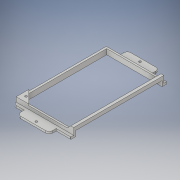
# Autodesk Inventor part: display_mount
Saved by Autodesk Inventor 2019 (Build 230136000, 136)
## iProperties
Created: 2021-12-03
Part Number: display_mount
Material: Generisch
Document SubType Name: Modeling
Designer: Bergi
Density: 1 g/cm^3
Appearance: Vorgabe
Author: Bergi
Autodesk Inventor part; units mm, degrees
ref_plane "YZ Plane" through (0, 0, 0) normal (1, 0, 0) x (0, 1, 0)
ref_plane "XZ Plane" through (0, 0, 0) normal (0, 1, 0) x (-1, 0, 0)
ref_plane "XY Plane" through (0, 0, 0) normal (0, 0, 1) x (1, 0, 0)
sketch "Skizze1" plane through (0, 0, 0) normal (0, 1, 0) x (-1, 0, 0)
  line L0 (-39, 60.5) -> (39, 60.5)
  line L1 (39, 60.5) -> (39, -60.5)
  line L2 (39, -60.5) -> (-39, -60.5)
  line L3 (-39, -60.5) -> (-39, 60.5)
  line L4 (-39, 60.5) -> (39, -60.5) construction
  line L5 (39, 60.5) -> (-39, -60.5) construction
  line L6 (42, 63.5) -> (-42, 63.5)
  line L7 (-42, 63.5) -> (-42, -63.5)
  line L8 (-42, -63.5) -> (42, -63.5)
  line L9 (42, -63.5) -> (42, 63.5)
  point P0 (0, 0)
  dimension "d0" = 78
  dimension "d1" = 121
  dimension "d2" = 3
  constraints: 20 end point, 4 parallel, 2 midpoint, 2 perpendicular, 1 horizontal, 3 other
  measures "d0" distance of L1.end L2.end
  measures "d1" distance of L0.end L1.end
  measures "d2" distance between parallel lines of L0 L6
extrude "Extrusion1" add sketch "Skizze1" along normal blind 7.5
sketch "Skizze2" plane through (0, 7.5, 0) normal (0, 1, 0) x (1, 0, 0)
  line L0 (39, -60.5) -> (-39, -60.5) projected
  line L1 (-39, -60.5) -> (-39, 60.5) projected
  circle A0 centre (-35.5, -56) radius 1.5
  point P0 (0, 0)
  dimension "d5" = 4.5
  dimension "d6" = 3.5
  dimension "d12" = 3
  constraints: 1 centre point, 1 coincident
  measures "d5" distance from line of L0 point (-35.5, -56)
  measures "d6" distance from line of L1 point (-35.5, -56)
  measures "d12" diameter of A0
sketch "Skizze3" plane through (0, 7.5, 0) normal (0, 1, 0) x (1, 0, 0)
  line L0 (-42, -63.5) -> (42, -63.5) projected
  line L1 (-42, -63.5) -> (-24, -63.5)
  line L2 (-42, -63.5) -> (-42, -45.5)
  line L3 (-42, 63.5) -> (-42, -63.5) projected
  line L4 (-42, -45.5) -> (-24, -63.5)
  point P0 (0, 0)
  dimension "d7" = 18
  dimension "d9" = 18
  constraints: 6 end point, 2 point on line
  measures "d7" distance of L0.start L1.end
  measures "d9" distance of L0.start L2.end
extrude "Extrusion2" add sketch "Skizze3" along normal blind 2
extrude "Extrusion3" cut sketch "Skizze2" along normal through all
ref_plane "Arbeitsebene1" through (0, 0, -60.5) normal (1, 0, 0) x (0, 0, -1)
ref_plane "Arbeitsebene2" through (39, 0, 0) normal (0, 0, -1) x (-1, 0, 0)
sketch "Skizze4" plane through (0, 0, 0) normal (0, -1, 0) x (1, 0, 0)
  line L0 (-39, -60.5) -> (-39, 60.5) projected
  line L1 (-39, 60.5) -> (39, 60.5) projected
  line L2 (39, 60.5) -> (39, -60.5) projected
  line L3 (39, -60.5) -> (-39, -60.5) projected
  line L4 (-42, 63.5) -> (42, 63.5) projected
  line L5 (-42, -63.5) -> (-42, 63.5) projected
  line L6 (42, -63.5) -> (-42, -63.5) projected
  line L7 (42, 63.5) -> (42, -63.5) projected
  line L8 (-42, 63.5) -> (42, 63.5) projected
  line L9 (-58.8, 0) -> (58.8, 0) construction
  line L10 (18.5, 63.5) -> (18.5, 72.5)
  line L11 (13.5, 77.5) -> (-21.5, 77.5)
  line L12 (-26.5, 72.5) -> (-26.5, 63.5)
  line L13 (42, 63.5) -> (42, 63.5)
  line L14 (38, 67.5) -> (-38, 67.5)
  line L15 (-42, 63.5) -> (-42, 63.5)
  line L16 (42, -63.5) -> (42, -63.5)
  line L17 (38, -67.5) -> (-38, -67.5)
  line L18 (-42, -63.5) -> (-42, -63.5)
  arc A0 (42, 63.5) -> (38, 67.5) centre (38, 63.5) ccw
  arc A1 (-38, 67.5) -> (-42, 63.5) centre (-38, 63.5) ccw
  arc A2 (-42, -63.5) -> (-38, -67.5) centre (-38, -63.5) ccw
  arc A3 (38, -67.5) -> (42, -63.5) centre (38, -63.5) ccw
  arc A4 (18.5, 72.5) -> (13.5, 77.5) centre (13.5, 72.5) ccw
  arc A5 (-21.5, 77.5) -> (-26.5, 72.5) centre (-21.5, 72.5) ccw
  line L19 (18.5, -63.5) -> (18.5, -72.5)
  line L20 (13.5, -77.5) -> (-21.5, -77.5)
  line L21 (-26.5, -72.5) -> (-26.5, -63.5)
  arc A6 (13.5, -77.5) -> (18.5, -72.5) centre (13.5, -72.5) ccw
  arc A7 (-26.5, -72.5) -> (-21.5, -77.5) centre (-21.5, -72.5) ccw
  line L22 (18.5, -63.5) -> (-26.5, -63.5)
  line L23 (42, -63.5) -> (-42, -63.5) projected
  line L24 (0, -109.9497) -> (0, 109.9497) construction
  point P0 (0, 0)
  point P1 (18.5, 77.5)
  point P2 (-26.5, 77.5)
  point P3 (-4, 77.5)
  point P4 (42, 67.5)
  point P5 (-42, 67.5)
  point P6 (42, -67.5)
  point P7 (-42, -67.5)
  point P8 (18.5, -77.5)
  point P9 (-26.5, -77.5)
  point P10 (-4, -77.5)
  point P11 (-4, 73)
  point P12 (-4, -73)
  dimension "d20" = 155
  dimension "d21" = 45
  dimension "d22" = 4
  dimension "d23" = 135
  dimension "d24" = 4
  dimension "d25" = 4
  dimension "d26" = 4
  dimension "d27" = 4
  dimension "d30" = 5
  dimension "d33" = 5.5
  constraints: 26 end point, 18 point on line, 16 point on circle, 14 symmetric about line, 12 tangent, 8 centre point, 5 perpendicular, 1 collinear, 1 equal radius, 1 midpoint, 1 vertical, 2 other
  measures "d20" diameter of L11 L9
  measures "d21" distance of point (18.5, 77.5) point (-26.5, 77.5)
  measures "d22" horizontal distance of point (0, 0) point (-4, 77.5)
  measures "d23" distance between parallel lines of L14 L17
  measures "d24" radius of A0
  measures "d25" radius of A1
  measures "d26" radius of A2
  measures "d27" radius of A3
  measures "d30" radius of A4
  measures "d33" distance from line of L14 point (-4, 73)
extrude "Extrusion4" add sketch "Skizze4" against normal blind 3 contours A1 L14 L12 L4 | L12 L14 L10 L4 | L6 L21 L17 A2 | L10 L14 A0 L4 | L6 L19 L17 L21 | L6 A3 L17 L19
extrude "Extrusion5" add sketch "Skizze4" against normal up to surface (3 mm away) contours L12 L14 L10 L4 | L12 A5 L11 A4 L10 L14 | L6 L19 L17 L21 | L17 L19 A6 L20 A7 L21
hole "Bohrung1" at (-4, 0, 73) at (-4, 0, -73) direction (0, 1, 0) diameter 3 end through all
sketch "Skizze6" plane through (42, 7.5, 63.5) normal (1, 0, 0) x (0, 0, -1)
  line L0 (0, -7.5) -> (127, -7.5) projected
  line L1 (127, -7.5) -> (127, -4.5) projected
  line L2 (127, -4.5) -> (127, 0) projected
  line L3 (0, 0) -> (127, 0) projected
  line L4 (0, -4.5) -> (0, 0) projected
  line L5 (0, -7.5) -> (0, -4.5) projected
  line L6 (131, -7.5) -> (127, -7.5) projected
  line L7 (131, -7.5) -> (131, -4.5) projected
  line L8 (127, -4.5) -> (131, -4.5) projected
  line L9 (127, -7.5) -> (127, -4.5) projected
  line L10 (0, -7.5) -> (-4, -7.5) projected
  line L11 (0, -7.5) -> (0, -4.5) projected
  line L12 (-4, -4.5) -> (0, -4.5) projected
  line L13 (-4, -7.5) -> (-4, -4.5) projected
  point P0 (63.5, -7.5)
extrude "Extrusion8" cut sketch "Skizze6" against normal up to surface (3 mm away)
sketch "Skizze7" plane through (0, 7.5, 0) normal (0, 1, 0) x (1, 0, 0)
  line L0 (39, -63.5) -> (39, -60.5) projected
  line L1 (39, -60.5) -> (-27, -60.5) projected
  line L2 (-27, -60.5) -> (-24, -63.5) projected
  line L3 (-24, -63.5) -> (39, -63.5) projected
  line L4 (39, 60.5) -> (39, 63.5) projected
  line L5 (39, 63.5) -> (-42, 63.5) projected
  line L6 (-42, 63.5) -> (-42, -45.5) projected
  line L7 (-42, -45.5) -> (-39, -48.5) projected
  line L8 (-39, -48.5) -> (-39, 60.5) projected
  line L9 (-39, 60.5) -> (39, 60.5) projected
  line L10 (39, -63.5) -> (39, 63.5)
  line L11 (39, 63.5) -> (-42, 63.5) projected
  line L12 (39, 63.5) -> (35, 63.5)
  line L13 (35, 63.5) -> (35, -63.5)
  line L14 (-42, -63.5) -> (39, -63.5) projected
  line L15 (35, -63.5) -> (39, -63.5)
  point P0 (0, 0)
  dimension "d48" = 4
  constraints: 8 end point, 2 collinear, 2 point on line, 1 perpendicular
  measures "d48" distance between parallel lines of L13 L10
extrude "Extrusion9" add sketch "Skizze7" along normal blind 5 contours L3 L13 L1 L0 | L1 L13 L9 L10 | L9 L13 L5 L4
sketch "Skizze8" plane through (-42, 3, -63.5) normal (0, 0, -1) x (-1, 0, 0)
  line L0 (-81, 9.5) -> (-81, 0) projected
  line L1 (-81, 0) -> (0, 0) projected
  line L2 (0, 0) -> (0, 4.5) projected
  line L3 (-77, 4.5) -> (0, 4.5) projected
  line L4 (-77, 4.5) -> (-77, 9.5) projected
  line L5 (-81, 9.5) -> (-77, 9.5) projected
  line L6 (-77, 4.5) -> (-77, 9.5) projected
  line L7 (-77, 9.5) -> (-72, 4.5)
  line L8 (-77, 4.5) -> (-15, 4.5) projected
  line L9 (-77, 9.5) -> (-69.9289, 9.5) construction
  line L10 (-72, 4.5) -> (-77, 4.5)
  line L11 (-77, 4.5) -> (-77, 9.5)
  point P0 (-42, -3)
  dimension "d51" = 45
  constraints: 8 end point, 1 collinear, 1 equal length, 1 horizontal, 1 perpendicular, 1 point on line
  measures "d51" angle of L7 L9
extrude "Extrusion10" add sketch "Skizze8" against normal up to surface (3 mm away) contours L7 L3 L4
sketch "Skizze9" plane through (-42, 9.5, 63.5) normal (0, 0, 1) x (1, 0, 0)
  line L0 (81, -9.5) -> (3, -9.5) projected
  line L1 (81, -9.5) -> (81, -2) projected
  line L2 (77, -2) -> (81, -2) projected
  line L3 (77, 3) -> (77, -2) projected
  line L4 (77, 3) -> (72, -2) projected
  line L5 (3, -2) -> (72, -2) projected
  line L6 (3, -9.5) -> (3, -2) projected
  line L7 (18, -2) -> (77, -2) projected
  line L8 (72, -2) -> (77, -2)
  point P0 (42, -9.5)
  constraints: 2 end point, 1 collinear
extrude "Extrusion11" add sketch "Skizze9" against normal up to surface (3 mm away) contours L7 L4 L3
sketch "Skizze10" plane through (0, 0, 0) normal (0, -1, 0) x (1, 0, 0)
  line L0 (39, -67.373) -> (39, -60.5) projected
  line L1 (39, -60.5) -> (-39, -60.5) projected
  line L2 (-39, -60.5) -> (-39, 60.5) projected
  line L3 (-39, 60.5) -> (39, 60.5) projected
  line L4 (39, 60.5) -> (39, 67.373) projected
  arc A0 (39, 67.373) -> (38, 67.5) centre (38, 63.5) ccw projected
  line L5 (38, 67.5) -> (18.5, 67.5) projected
  line L6 (18.5, 67.5) -> (18.5, 72.5) projected
  arc A1 (18.5, 72.5) -> (13.5, 77.5) centre (13.5, 72.5) ccw projected
  line L7 (13.5, 77.5) -> (-21.5, 77.5) projected
  arc A2 (-21.5, 77.5) -> (-26.5, 72.5) centre (-21.5, 72.5) ccw projected
  line L8 (-26.5, 72.5) -> (-26.5, 67.5) projected
  line L9 (-26.5, 67.5) -> (-38, 67.5) projected
  arc A3 (-38, 67.5) -> (-42, 63.5) centre (-38, 63.5) ccw projected
  line L10 (-42, -63.5) -> (-42, 63.5) projected
  arc A4 (-42, -63.5) -> (-38, -67.5) centre (-38, -63.5) ccw projected
  line L11 (-38, -67.5) -> (-26.5, -67.5) projected
  line L12 (-26.5, -67.5) -> (-26.5, -72.5) projected
  arc A5 (-26.5, -72.5) -> (-21.5, -77.5) centre (-21.5, -72.5) ccw projected
  line L13 (-21.5, -77.5) -> (13.5, -77.5) projected
  arc A6 (13.5, -77.5) -> (18.5, -72.5) centre (13.5, -72.5) ccw projected
  line L14 (18.5, -72.5) -> (18.5, -67.5) projected
  line L15 (18.5, -67.5) -> (38, -67.5) projected
  arc A7 (38, -67.5) -> (39, -67.373) centre (38, -63.5) ccw projected
  circle A8 centre (-4, -73) radius 1.5 projected
  circle A9 centre (-4, 73) radius 1.5 projected
  line L16 (39, 61) -> (-39, 61)
  line L17 (-39, -60.5) -> (-39, 60.5) projected
  line L18 (-39, 60.5) -> (-39, 61)
  line L19 (39, -61) -> (-39, -61)
  line L20 (-39, -61) -> (-39, -60.5)
  point P0 (0, 0)
  dimension "d56" = 0.5
  dimension "d57" = 0.5
  constraints: 8 end point, 3 point on line, 1 parallel, 1 perpendicular, 1 vertical
  measures "d56" distance between parallel lines of L3 L16
  measures "d57" distance between parallel lines of L19 L1
extrude "Extrusion12" cut sketch "Skizze10" against normal up to surface (7.5 mm away) contours L19 L20 L1 L0 | L18 L16 L4 L3
